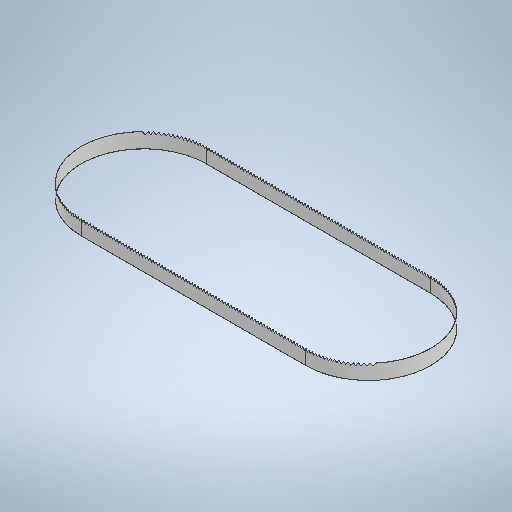
# Autodesk Inventor part: Saw
Saved by Autodesk Inventor 2025.2 (Build 292293000, 293)
## iProperties
Created: 2025-05-26
Part Number: Saw
Material: Generic
Document SubType Name: Modeling
Designer: abdal
Density: 1 g/cm^3
Appearance: Default
Author: abdal
Autodesk Inventor part; units mm, degrees
ref_plane "YZ Plane" through (0, 0, 0) normal (1, 0, 0) x (0, 1, 0)
ref_plane "XZ Plane" through (0, 0, 0) normal (0, 1, 0) x (-1, 0, 0)
ref_plane "XY Plane" through (0, 0, 0) normal (0, 0, 1) x (1, 0, 0)
sketch "Sketch1" plane through (0, 0, 0) normal (0, 1, 0) x (-1, 0, 0)
  line L0 (1125, 0) -> (-1125, 0) construction
  line L1 (1125, 625) -> (-1125, 625)
  line L2 (-1125, -625) -> (1125, -625)
  arc A0 (1125, -625) -> (1125, 625) centre (1125, 0) ccw
  arc A1 (-1125, 625) -> (-1125, -625) centre (-1125, 0) ccw
  line L3 (-1125, 626.25) -> (1125, 626.25)
  arc A2 (1125, -626.25) -> (1125, 626.25) centre (1125, 0) ccw
  line L4 (1125, -626.25) -> (-1125, -626.25)
  arc A3 (-1125, 626.25) -> (-1125, -626.25) centre (-1125, 0) ccw
  point P0 (0, 0)
  point P1 (0, 0)
  dimension "d0" = 2250
  dimension "d1" = 1250
  dimension "d2" = 1.25
  constraints: 12 end point, 8 point on circle, 4 centre point, 4 tangent, 2 parallel, 1 coincident, 1 horizontal, 1 midpoint, 3 other
  measures "d0" distance of L0.start L0.end
  measures "d1" distance of L2.end L1.start
  measures "d2" distance between parallel lines of L1 L3
extrude "Extrusion1" add sketch "Sketch1" along normal blind 150
sketch "Sketch2" plane through (-1125, 0, 626.25) normal (0, 0, 1) x (1, 0, 0)
  line L0 (0, 0) -> (2250, 0) projected
  line L1 (2250, 0) -> (2250, 150) projected
  line L2 (0, 150) -> (2250, 150) projected
  line L3 (0, 0) -> (0, 150) projected
  line L4 (0, 0) -> (0, 0) projected
  line L5 (0, 0) -> (0, 150) projected
  line L6 (0, 150) -> (0, 150) projected
  line L7 (0, 0) -> (0, 150) projected
  line L8 (2250, 0) -> (2250, 0) projected
  line L9 (2250, 0) -> (2250, 150) projected
  line L10 (2250, 150) -> (2250, 150) projected
  line L11 (2250, 0) -> (2250, 150) projected
  line L12 (0, 150) -> (30, 150)
  line L13 (30, 150) -> (15, 124.0192)
  line L14 (15, 124.0192) -> (0, 150)
  line L15 (60, 150) -> (45, 124.0192)
  line L16 (30, 150) -> (60, 150)
  line L17 (45, 124.0192) -> (30, 150)
  line L18 (90, 150) -> (75, 124.0192)
  line L19 (60, 150) -> (90, 150)
  line L20 (75, 124.0192) -> (60, 150)
  line L21 (120, 150) -> (105, 124.0192)
  line L22 (90, 150) -> (120, 150)
  line L23 (105, 124.0192) -> (90, 150)
  line L24 (150, 150) -> (135, 124.0192)
  line L25 (120, 150) -> (150, 150)
  line L26 (135, 124.0192) -> (120, 150)
  line L27 (180, 150) -> (165, 124.0192)
  line L28 (150, 150) -> (180, 150)
  line L29 (165, 124.0192) -> (150, 150)
  line L30 (210, 150) -> (195, 124.0192)
  line L31 (180, 150) -> (210, 150)
  line L32 (195, 124.0192) -> (180, 150)
  line L33 (240, 150) -> (225, 124.0192)
  line L34 (210, 150) -> (240, 150)
  line L35 (225, 124.0192) -> (210, 150)
  line L36 (270, 150) -> (255, 124.0192)
  line L37 (240, 150) -> (270, 150)
  line L38 (255, 124.0192) -> (240, 150)
  line L39 (300, 150) -> (285, 124.0192)
  line L40 (270, 150) -> (300, 150)
  line L41 (285, 124.0192) -> (270, 150)
  line L42 (330, 150) -> (315, 124.0192)
  line L43 (300, 150) -> (330, 150)
  line L44 (315, 124.0192) -> (300, 150)
  line L45 (360, 150) -> (345, 124.0192)
  line L46 (330, 150) -> (360, 150)
  line L47 (345, 124.0192) -> (330, 150)
  line L48 (390, 150) -> (375, 124.0192)
  line L49 (360, 150) -> (390, 150)
  line L50 (375, 124.0192) -> (360, 150)
  line L51 (420, 150) -> (405, 124.0192)
  line L52 (390, 150) -> (420, 150)
  line L53 (405, 124.0192) -> (390, 150)
  line L54 (450, 150) -> (435, 124.0192)
  line L55 (420, 150) -> (450, 150)
  line L56 (435, 124.0192) -> (420, 150)
  line L57 (480, 150) -> (465, 124.0192)
  line L58 (450, 150) -> (480, 150)
  line L59 (465, 124.0192) -> (450, 150)
  line L60 (510, 150) -> (495, 124.0192)
  line L61 (480, 150) -> (510, 150)
  line L62 (495, 124.0192) -> (480, 150)
  line L63 (540, 150) -> (525, 124.0192)
  line L64 (510, 150) -> (540, 150)
  line L65 (525, 124.0192) -> (510, 150)
  line L66 (570, 150) -> (555, 124.0192)
  line L67 (540, 150) -> (570, 150)
  line L68 (555, 124.0192) -> (540, 150)
  line L69 (600, 150) -> (585, 124.0192)
  line L70 (570, 150) -> (600, 150)
  line L71 (585, 124.0192) -> (570, 150)
  line L72 (630, 150) -> (615, 124.0192)
  line L73 (600, 150) -> (630, 150)
  line L74 (615, 124.0192) -> (600, 150)
  line L75 (660, 150) -> (645, 124.0192)
  line L76 (630, 150) -> (660, 150)
  line L77 (645, 124.0192) -> (630, 150)
  line L78 (690, 150) -> (675, 124.0192)
  line L79 (660, 150) -> (690, 150)
  line L80 (675, 124.0192) -> (660, 150)
  line L81 (720, 150) -> (705, 124.0192)
  line L82 (690, 150) -> (720, 150)
  line L83 (705, 124.0192) -> (690, 150)
  line L84 (750, 150) -> (735, 124.0192)
  line L85 (720, 150) -> (750, 150)
  line L86 (735, 124.0192) -> (720, 150)
  line L87 (780, 150) -> (765, 124.0192)
  line L88 (750, 150) -> (780, 150)
  line L89 (765, 124.0192) -> (750, 150)
  line L90 (810, 150) -> (795, 124.0192)
  line L91 (780, 150) -> (810, 150)
  line L92 (795, 124.0192) -> (780, 150)
  line L93 (840, 150) -> (825, 124.0192)
  line L94 (810, 150) -> (840, 150)
  line L95 (825, 124.0192) -> (810, 150)
  line L96 (870, 150) -> (855, 124.0192)
  line L97 (840, 150) -> (870, 150)
  line L98 (855, 124.0192) -> (840, 150)
  line L99 (900, 150) -> (885, 124.0192)
  line L100 (870, 150) -> (900, 150)
  line L101 (885, 124.0192) -> (870, 150)
  line L102 (930, 150) -> (915, 124.0192)
  line L103 (900, 150) -> (930, 150)
  line L104 (915, 124.0192) -> (900, 150)
  line L105 (960, 150) -> (945, 124.0192)
  line L106 (930, 150) -> (960, 150)
  line L107 (945, 124.0192) -> (930, 150)
  line L108 (990, 150) -> (975, 124.0192)
  line L109 (960, 150) -> (990, 150)
  line L110 (975, 124.0192) -> (960, 150)
  line L111 (1020, 150) -> (1005, 124.0192)
  line L112 (990, 150) -> (1020, 150)
  line L113 (1005, 124.0192) -> (990, 150)
  line L114 (1050, 150) -> (1035, 124.0192)
  line L115 (1020, 150) -> (1050, 150)
  line L116 (1035, 124.0192) -> (1020, 150)
  line L117 (1080, 150) -> (1065, 124.0192)
  line L118 (1050, 150) -> (1080, 150)
  line L119 (1065, 124.0192) -> (1050, 150)
  line L120 (1110, 150) -> (1095, 124.0192)
  line L121 (1080, 150) -> (1110, 150)
  line L122 (1095, 124.0192) -> (1080, 150)
  line L123 (1140, 150) -> (1125, 124.0192)
  line L124 (1110, 150) -> (1140, 150)
  line L125 (1125, 124.0192) -> (1110, 150)
  line L126 (1170, 150) -> (1155, 124.0192)
  line L127 (1140, 150) -> (1170, 150)
  line L128 (1155, 124.0192) -> (1140, 150)
  line L129 (1200, 150) -> (1185, 124.0192)
  line L130 (1170, 150) -> (1200, 150)
  line L131 (1185, 124.0192) -> (1170, 150)
  line L132 (1230, 150) -> (1215, 124.0192)
  line L133 (1200, 150) -> (1230, 150)
  line L134 (1215, 124.0192) -> (1200, 150)
  line L135 (1260, 150) -> (1245, 124.0192)
  line L136 (1230, 150) -> (1260, 150)
  line L137 (1245, 124.0192) -> (1230, 150)
  line L138 (1290, 150) -> (1275, 124.0192)
  line L139 (1260, 150) -> (1290, 150)
  line L140 (1275, 124.0192) -> (1260, 150)
  line L141 (1320, 150) -> (1305, 124.0192)
  line L142 (1290, 150) -> (1320, 150)
  line L143 (1305, 124.0192) -> (1290, 150)
  line L144 (1350, 150) -> (1335, 124.0192)
  line L145 (1320, 150) -> (1350, 150)
  line L146 (1335, 124.0192) -> (1320, 150)
  line L147 (1380, 150) -> (1365, 124.0192)
  line L148 (1350, 150) -> (1380, 150)
  line L149 (1365, 124.0192) -> (1350, 150)
  line L150 (1410, 150) -> (1395, 124.0192)
  line L151 (1380, 150) -> (1410, 150)
  line L152 (1395, 124.0192) -> (1380, 150)
  line L153 (1440, 150) -> (1425, 124.0192)
  line L154 (1410, 150) -> (1440, 150)
  line L155 (1425, 124.0192) -> (1410, 150)
  line L156 (1470, 150) -> (1455, 124.0192)
  line L157 (1440, 150) -> (1470, 150)
  line L158 (1455, 124.0192) -> (1440, 150)
  line L159 (1500, 150) -> (1485, 124.0192)
  line L160 (1470, 150) -> (1500, 150)
  line L161 (1485, 124.0192) -> (1470, 150)
  line L162 (1530, 150) -> (1515, 124.0192)
  line L163 (1500, 150) -> (1530, 150)
  line L164 (1515, 124.0192) -> (1500, 150)
  line L165 (1560, 150) -> (1545, 124.0192)
  line L166 (1530, 150) -> (1560, 150)
  line L167 (1545, 124.0192) -> (1530, 150)
  line L168 (1590, 150) -> (1575, 124.0192)
  line L169 (1560, 150) -> (1590, 150)
  line L170 (1575, 124.0192) -> (1560, 150)
  line L171 (1620, 150) -> (1605, 124.0192)
  line L172 (1590, 150) -> (1620, 150)
  line L173 (1605, 124.0192) -> (1590, 150)
  line L174 (1650, 150) -> (1635, 124.0192)
  line L175 (1620, 150) -> (1650, 150)
  line L176 (1635, 124.0192) -> (1620, 150)
  line L177 (1680, 150) -> (1665, 124.0192)
  line L178 (1650, 150) -> (1680, 150)
  line L179 (1665, 124.0192) -> (1650, 150)
  line L180 (1710, 150) -> (1695, 124.0192)
  line L181 (1680, 150) -> (1710, 150)
  line L182 (1695, 124.0192) -> (1680, 150)
  line L183 (1740, 150) -> (1725, 124.0192)
  line L184 (1710, 150) -> (1740, 150)
  line L185 (1725, 124.0192) -> (1710, 150)
  line L186 (1770, 150) -> (1755, 124.0192)
  line L187 (1740, 150) -> (1770, 150)
  line L188 (1755, 124.0192) -> (1740, 150)
  line L189 (1800, 150) -> (1785, 124.0192)
  line L190 (1770, 150) -> (1800, 150)
  line L191 (1785, 124.0192) -> (1770, 150)
  line L192 (1830, 150) -> (1815, 124.0192)
  line L193 (1800, 150) -> (1830, 150)
  line L194 (1815, 124.0192) -> (1800, 150)
  line L195 (1860, 150) -> (1845, 124.0192)
  line L196 (1830, 150) -> (1860, 150)
  line L197 (1845, 124.0192) -> (1830, 150)
  line L198 (1890, 150) -> (1875, 124.0192)
  line L199 (1860, 150) -> (1890, 150)
  line L200 (1875, 124.0192) -> (1860, 150)
  line L201 (1920, 150) -> (1905, 124.0192)
  line L202 (1890, 150) -> (1920, 150)
  line L203 (1905, 124.0192) -> (1890, 150)
  line L204 (1950, 150) -> (1935, 124.0192)
  line L205 (1920, 150) -> (1950, 150)
  line L206 (1935, 124.0192) -> (1920, 150)
  line L207 (1980, 150) -> (1965, 124.0192)
  line L208 (1950, 150) -> (1980, 150)
  line L209 (1965, 124.0192) -> (1950, 150)
  line L210 (2010, 150) -> (1995, 124.0192)
  line L211 (1980, 150) -> (2010, 150)
  line L212 (1995, 124.0192) -> (1980, 150)
  line L213 (2040, 150) -> (2025, 124.0192)
  line L214 (2010, 150) -> (2040, 150)
  line L215 (2025, 124.0192) -> (2010, 150)
  line L216 (2070, 150) -> (2055, 124.0192)
  line L217 (2040, 150) -> (2070, 150)
  line L218 (2055, 124.0192) -> (2040, 150)
  line L219 (2100, 150) -> (2085, 124.0192)
  line L220 (2070, 150) -> (2100, 150)
  line L221 (2085, 124.0192) -> (2070, 150)
  line L222 (2130, 150) -> (2115, 124.0192)
  line L223 (2100, 150) -> (2130, 150)
  line L224 (2115, 124.0192) -> (2100, 150)
  line L225 (2160, 150) -> (2145, 124.0192)
  line L226 (2130, 150) -> (2160, 150)
  line L227 (2145, 124.0192) -> (2130, 150)
  line L228 (2190, 150) -> (2175, 124.0192)
  line L229 (2160, 150) -> (2190, 150)
  line L230 (2175, 124.0192) -> (2160, 150)
  line L231 (2220, 150) -> (2205, 124.0192)
  line L232 (2190, 150) -> (2220, 150)
  line L233 (2205, 124.0192) -> (2190, 150)
  line L234 (2250, 150) -> (2235, 124.0192)
  line L235 (2220, 150) -> (2250, 150)
  line L236 (2235, 124.0192) -> (2220, 150)
  line L237 (2280, 150) -> (2265, 124.0192)
  line L238 (2250, 150) -> (2280, 150)
  line L239 (2265, 124.0192) -> (2250, 150)
  line L240 (2310, 150) -> (2295, 124.0192)
  line L241 (2280, 150) -> (2310, 150)
  line L242 (2295, 124.0192) -> (2280, 150)
  line L243 (2340, 150) -> (2325, 124.0192)
  line L244 (2310, 150) -> (2340, 150)
  line L245 (2325, 124.0192) -> (2310, 150)
  line L246 (2370, 150) -> (2355, 124.0192)
  line L247 (2340, 150) -> (2370, 150)
  line L248 (2355, 124.0192) -> (2340, 150)
  line L249 (2400, 150) -> (2385, 124.0192)
  line L250 (2370, 150) -> (2400, 150)
  line L251 (2385, 124.0192) -> (2370, 150)
  line L252 (0, 150) -> (-15, 124.0192)
  line L253 (-15, 124.0192) -> (-30, 150)
  line L254 (-30, 150) -> (0, 150)
  line L255 (-30, 150) -> (-45, 124.0192)
  line L256 (-45, 124.0192) -> (-60, 150)
  line L257 (-60, 150) -> (-30, 150)
  line L258 (-60, 150) -> (-75, 124.0192)
  line L259 (-75, 124.0192) -> (-90, 150)
  line L260 (-90, 150) -> (-60, 150)
  line L261 (-90, 150) -> (-105, 124.0192)
  line L262 (-105, 124.0192) -> (-120, 150)
  line L263 (-120, 150) -> (-90, 150)
  line L264 (-120, 150) -> (-135, 124.0192)
  line L265 (-135, 124.0192) -> (-150, 150)
  line L266 (-150, 150) -> (-120, 150)
  line L267 (-150, 150) -> (-165, 124.0192)
  line L268 (-165, 124.0192) -> (-180, 150)
  line L269 (-180, 150) -> (-150, 150)
  line L270 (-180, 150) -> (-195, 124.0192)
  line L271 (-195, 124.0192) -> (-210, 150)
  line L272 (-210, 150) -> (-180, 150)
  line L273 (-210, 150) -> (-225, 124.0192)
  line L274 (-225, 124.0192) -> (-240, 150)
  line L275 (-240, 150) -> (-210, 150)
  line L276 (-240, 150) -> (-255, 124.0192)
  line L277 (-255, 124.0192) -> (-270, 150)
  line L278 (-270, 150) -> (-240, 150)
  line L279 (-270, 150) -> (-285, 124.0192)
  line L280 (-285, 124.0192) -> (-300, 150)
  line L281 (-300, 150) -> (-270, 150)
  line L282 (-300, 150) -> (-315, 124.0192)
  line L283 (-315, 124.0192) -> (-330, 150)
  line L284 (-330, 150) -> (-300, 150)
  line L285 (-330, 150) -> (-345, 124.0192)
  line L286 (-345, 124.0192) -> (-360, 150)
  line L287 (-360, 150) -> (-330, 150)
  line L288 (-360, 150) -> (-375, 124.0192)
  line L289 (-375, 124.0192) -> (-390, 150)
  line L290 (-390, 150) -> (-360, 150)
  line L291 (-390, 150) -> (-405, 124.0192)
  line L292 (-405, 124.0192) -> (-420, 150)
  line L293 (-420, 150) -> (-390, 150)
  line L294 (-420, 150) -> (-435, 124.0192)
  line L295 (-435, 124.0192) -> (-450, 150)
  line L296 (-450, 150) -> (-420, 150)
  line L297 (-450, 150) -> (-465, 124.0192)
  line L298 (-465, 124.0192) -> (-480, 150)
  line L299 (-480, 150) -> (-450, 150)
  line L300 (-480, 150) -> (-495, 124.0192)
  line L301 (-495, 124.0192) -> (-510, 150)
  line L302 (-510, 150) -> (-480, 150)
  line L303 (-510, 150) -> (-525, 124.0192)
  line L304 (-525, 124.0192) -> (-540, 150)
  line L305 (-540, 150) -> (-510, 150)
  line L306 (-540, 150) -> (-555, 124.0192)
  line L307 (-555, 124.0192) -> (-570, 150)
  line L308 (-570, 150) -> (-540, 150)
  line L309 (-570, 150) -> (-585, 124.0192)
  line L310 (-585, 124.0192) -> (-600, 150)
  line L311 (-600, 150) -> (-570, 150)
  line L312 (-600, 150) -> (-615, 124.0192)
  line L313 (-615, 124.0192) -> (-630, 150)
  line L314 (-630, 150) -> (-600, 150)
  line L315 (-630, 150) -> (-645, 124.0192)
  line L316 (-645, 124.0192) -> (-660, 150)
  line L317 (-660, 150) -> (-630, 150)
  line L318 (-660, 150) -> (-675, 124.0192)
  line L319 (-675, 124.0192) -> (-690, 150)
  line L320 (-690, 150) -> (-660, 150)
  line L321 (-690, 150) -> (-705, 124.0192)
  line L322 (-705, 124.0192) -> (-720, 150)
  line L323 (-720, 150) -> (-690, 150)
  line L324 (2430, 150) -> (2415, 124.0192)
  line L325 (2400, 150) -> (2430, 150)
  line L326 (2415, 124.0192) -> (2400, 150)
  line L327 (2460, 150) -> (2445, 124.0192)
  line L328 (2430, 150) -> (2460, 150)
  line L329 (2445, 124.0192) -> (2430, 150)
  line L330 (2490, 150) -> (2475, 124.0192)
  line L331 (2460, 150) -> (2490, 150)
  line L332 (2475, 124.0192) -> (2460, 150)
  line L333 (2520, 150) -> (2505, 124.0192)
  line L334 (2490, 150) -> (2520, 150)
  line L335 (2505, 124.0192) -> (2490, 150)
  line L336 (2550, 150) -> (2535, 124.0192)
  line L337 (2520, 150) -> (2550, 150)
  line L338 (2535, 124.0192) -> (2520, 150)
  line L339 (2580, 150) -> (2565, 124.0192)
  line L340 (2550, 150) -> (2580, 150)
  line L341 (2565, 124.0192) -> (2550, 150)
  line L342 (2610, 150) -> (2595, 124.0192)
  line L343 (2580, 150) -> (2610, 150)
  line L344 (2595, 124.0192) -> (2580, 150)
  line L345 (2640, 150) -> (2625, 124.0192)
  line L346 (2610, 150) -> (2640, 150)
  line L347 (2625, 124.0192) -> (2610, 150)
  line L348 (2670, 150) -> (2655, 124.0192)
  line L349 (2640, 150) -> (2670, 150)
  line L350 (2655, 124.0192) -> (2640, 150)
  line L351 (2700, 150) -> (2685, 124.0192)
  line L352 (2670, 150) -> (2700, 150)
  line L353 (2685, 124.0192) -> (2670, 150)
  line L354 (2730, 150) -> (2715, 124.0192)
  line L355 (2700, 150) -> (2730, 150)
  line L356 (2715, 124.0192) -> (2700, 150)
  line L357 (2760, 150) -> (2745, 124.0192)
  line L358 (2730, 150) -> (2760, 150)
  line L359 (2745, 124.0192) -> (2730, 150)
  line L360 (2790, 150) -> (2775, 124.0192)
  line L361 (2760, 150) -> (2790, 150)
  line L362 (2775, 124.0192) -> (2760, 150)
  line L363 (2820, 150) -> (2805, 124.0192)
  line L364 (2790, 150) -> (2820, 150)
  line L365 (2805, 124.0192) -> (2790, 150)
  line L366 (2850, 150) -> (2835, 124.0192)
  line L367 (2820, 150) -> (2850, 150)
  line L368 (2835, 124.0192) -> (2820, 150)
  line L369 (2880, 150) -> (2865, 124.0192)
  line L370 (2850, 150) -> (2880, 150)
  line L371 (2865, 124.0192) -> (2850, 150)
  line L372 (2910, 150) -> (2895, 124.0192)
  line L373 (2880, 150) -> (2910, 150)
  line L374 (2895, 124.0192) -> (2880, 150)
  point P0 (1125, 0)
  point P1 (2300, 150)
  point P2 (630, 150)
  point P3 (630, 150)
  point P4 (630, 150)
  point P5 (600, 150)
  point P6 (600, 150)
  point P7 (600, 150)
  point P8 (570, 150)
  point P9 (570, 150)
  point P10 (570, 150)
  point P11 (540, 150)
  point P12 (540, 150)
  point P13 (540, 150)
  point P14 (2300, 132.6795)
  dimension "d5" = 30
  dimension "d6" = 30
  dimension "d7" = 30
  dimension "d10" = 30
  dimension "d22" = 30
  constraints: 726 end point, 384 horizontal alignment, 240 parallel, 120 collinear, 1 horizontal
  measures "d5" distance of L12.end L13.end
  measures "d6" distance of L3.end L12.end
  measures "d7" distance of L3.end L13.end
  measures "d10" distance of L12.end L15.start
  measures "d22" distance of L13.end L252.end
extrude "Extrusion2" cut sketch "Sketch2" against normal through all contours L321 L322 L323 | L318 L319 L320 | L315 L316 L317 | L294 L295 L296 | L291 L292 L293 | L288 L289 L290 | L285 L286 L287 | L282 L283 L284 | L279 L280 L281 | L276 L277 L278 | L273 L274 L275 | L270 L271 L272 | L267 L268 L269 | L264 L265 L266 | L261 L262 L263 | L258 L259 L260 | L255 L256 L257 | L252 L253 L254 | L355 L354 L356 | L352 L351 L353 | L349 L348 L350 | L346 L345 L347 | L343 L342 L344 | L340 L339 L341 | L337 L336 L338 | L334 L333 L335 | L331 L330 L332 | L328 L327 L329 | L325 L324 L326 | L250 L249 L251 | L247 L246 L248 | L244 L243 L245 | L241 L240 L242 | L238 L237 L239 | L2 L13 L14 | L234 L236 L2 | L2 L15 L17 | L231 L233 L2 | L2 L18 L20 | L228 L230 L2 | L2 L21 L23 | L225 L227 L2 | L2 L24 L26 | L222 L224 L2 | L2 L27 L29 | L219 L221 L2 | L2 L30 L32 | L216 L218 L2 | L2 L33 L35 | L213 L215 L2 | L2 L36 L38 | L210 L212 L2 | L2 L39 L41 | L207 L209 L2 | L2 L42 L44 | L204 L206 L2 | L2 L45 L47 | L201 L203 L2 | L2 L48 L50 | L198 L200 L2 | L2 L51 L53 | L195 L197 L2 | L2 L54 L56 | L192 L194 L2 | L2 L57 L59 | L189 L191 L2 | L2 L60 L62 | L186 L188 L2 | L2 L63 L65 | L183 L185 L2 | L2 L66 L68 | L180 L182 L2 | L2 L69 L71 | L177 L179 L2 | L2 L72 L74 | L174 L176 L2 | L2 L75 L77 | L171 L173 L2 | L2 L78 L80 | L168 L170 L2 | L2 L81 L83 | L165 L167 L2 | L2 L84 L86 | L162 L164 L2 | L2 L87 L89 | L159 L161 L2 | L2 L90 L92 | L156 L158 L2 | L2 L93 L95 | L153 L155 L2 | L2 L96 L98 | L150 L152 L2 | L2 L99 L101 | L147 L149 L2 | L2 L102 L104 | L144 L146 L2 | L2 L105 L107 | L141 L143 L2 | L2 L108 L110 | L138 L140 L2 | L2 L111 L113 | L135 L137 L2 | L2 L114 L116 | L132 L134 L2 | L2 L117 L119 | L129 L131 L2 | L2 L120 L122 | L126 L128 L2 | L2 L123 L125
body "Solid1"
